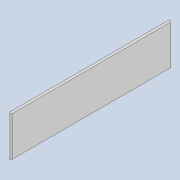
# Autodesk Inventor part: fin_12mm
Saved by Autodesk Inventor 2020 (Build 240168000, 168)
## iProperties
Created: 2021-10-03
Part Number: fin_12mm
Material: Generic
Document SubType Name: Modeling
Designer: Shuang Peng
Density: 1 g/cm^3
Appearance: Default
Author: Shuang Peng
Autodesk Inventor part; units mm, degrees
ref_plane "YZ Plane" through (0, 0, 0) normal (1, 0, 0) x (0, 1, 0)
ref_plane "XZ Plane" through (0, 0, 0) normal (0, 1, 0) x (-1, 0, 0)
ref_plane "XY Plane" through (0, 0, 0) normal (0, 0, 1) x (1, 0, 0)
sketch "Sketch1" plane through (0, 0, 0) normal (0, 1, 0) x (-1, 0, 0)
  line L0 (0, 0) -> (0, -12) construction
  line L1 (-0.1, 0) -> (-0.1, -12)
  line L2 (0.1, -12) -> (0.1, 0)
  arc A0 (0.1, 0) -> (-0.1, 0) centre (0, 0) ccw
  arc A1 (-0.1, -12) -> (0.1, -12) centre (0, -12) ccw
  point P0 (0, -6)
  dimension "d0" = 12
  dimension "d1" = 0.2
  constraints: 8 end point, 4 point on circle, 4 tangent, 2 centre point, 1 midpoint, 1 parallel, 1 vertical
  measures "d0" distance of L0.start L0.end
  measures "d1" diameter of A1
extrude "Extrusion1" add sketch "Sketch1" along normal blind 3
body "Solid1"
